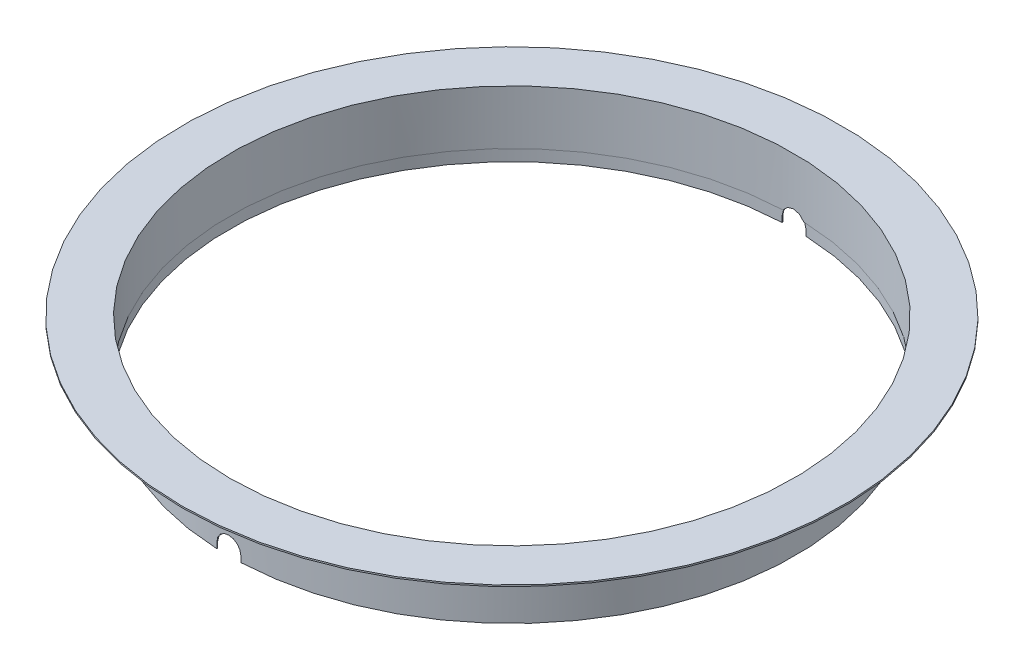
# Autodesk Inventor part: Layer2_Top
Saved by Autodesk Inventor 2017 (Build 210142000, 142)
## iProperties
Created: 2016-12-23
Part Number: Layer2_Top
Material: Generic
Document SubType Name: Modeling
Designer: David Kopala
Density: 1 g/cm^3
Appearance: Default
Author: David Kopala
Autodesk Inventor part; units mm, degrees
ref_plane "YZ Plane" through (0, 0, 0) normal (1, 0, 0) x (0, 1, 0)
ref_plane "XZ Plane" through (0, 0, 0) normal (0, 1, 0) x (-1, 0, 0)
sketch "Sketch1" plane through (0, 0, 0) normal (1, 0, 0) x (0, 1, 0)
  line L0 (0, 0) -> (0.4853, 0)
  line L1 (3.175, 149.225) -> (31.9024, 149.225)
  line L2 (31.9024, 149.225) -> (31.9024, 174.625)
  line L3 (31.9024, 174.625) -> (31.1086, 174.625)
  line L4 (31.1086, 174.625) -> (31.1087, 150.0187)
  line L5 (31.1087, 150.0187) -> (3.175, 150.0187)
  line L6 (0, 149.225) -> (-3.175, 149.225)
  line L7 (-3.175, 149.6219) -> (3.175, 149.6219)
  line L8 (3.175, 150.0187) -> (-3.175, 150.0187)
  line L9 (-3.175, 150.0187) -> (-3.175, 149.6219)
  line L10 (3.175, 149.6219) -> (3.175, 149.225)
  point P0 (31.4127, 174.625)
  dimension "d0" = 31.9024
  dimension "d1" = 149.225
  dimension "d2" = 25.4
  dimension "d3" = 0.7937
  dimension "d4" = 24.6062
  dimension "d5" = 3.175
  dimension "d6" = 0.3969
  constraints: 22 end point, 5 perpendicular, 2 horizontal, 1 parallel, 1 point on line, 1 vertical
  measures "d0" distance of L6.start L1.end
  measures "d1" distance between parallel lines of L0 L1
  measures "d2" distance of L1.end L2.end
  measures "d3" distance of L2.end L3.end
  measures "d4" distance of L3.end L4.end
  measures "d5" distance of L6.start L6.end
  measures "d6" distance of L6.end L7.start
revolve "Revolution1" add sketch "Sketch1" angle 360 about axis through (0, 0, 0) along (0, 1, 0)
ref_plane "Work Plane1" through (0, 31.4127, 174.625) normal (0, 0, 1) x (1, 0, 0)
sketch "Sketch2" plane through (0, 31.4127, 174.625) normal (0, 0, 1) x (1, 0, 0)
  line L0 (149.6219, -34.5877) -> (-149.6219, -34.5877) projected
  arc A0 (6.35, -31.4127) -> (-6.35, -31.4127) centre (0, -31.4127) ccw
  line L1 (-6.35, -34.5877) -> (-6.35, -31.4127)
  line L2 (6.35, -34.5877) -> (6.35, -31.4127)
  line L3 (-6.35, -34.5877) -> (6.35, -34.5877)
  point P0 (0, -31.4127)
  dimension "d10" = 12.7
  dimension "d11" = 0
  dimension "d12" = 3.175
  constraints: 6 end point, 2 point on circle, 2 point on line, 2 tangent, 1 centre point, 1 collinear
  measures "d10" diameter of A0
  measures "d11" distance of point (0, -31.413) A0.centre
  measures "d12" distance from line of L0 A0.centre
extrude "Extrusion1" cut sketch "Sketch2" against normal through all
body "Solid1"
